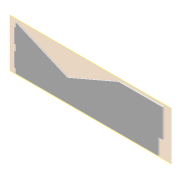
# Autodesk Inventor part: Frontal
Saved by Autodesk Inventor 2022 (Build 260153000, 153)
## iProperties
Created: 2022-06-06
Part Number: Frontal
Material: Generic
Document SubType Name: Modeling
Designer: ADMIN
Density: 1 g/cm^3
Appearance: Default
Author: ADMIN
Autodesk Inventor part; units mm, degrees
ref_plane "YZ Plane" through (0, 0, 0) normal (1, 0, 0) x (0, 1, 0)
ref_plane "XZ Plane" through (0, 0, 0) normal (0, 1, 0) x (-1, 0, 0)
ref_plane "XY Plane" through (0, 0, 0) normal (0, 0, 1) x (1, 0, 0)
ref_plane "Work Plane1" through (-2241.136, -81.6179, 0) normal (0, 0, 1) x (1, 0, 0)
sketch "Sketch1" plane through (-2241.136, -81.6179, 0) normal (0, 0, 1) x (1, 0, 0)
  line L0 (2006.136, 61.2134) -> (2006.136, 6.6179) projected
  line L1 (2006.136, 6.6179) -> (2476.136, 6.6179) projected
  line L2 (2476.136, 6.6179) -> (2476.136, 61.2134) projected
  line L3 (2476.136, 61.2134) -> (2491.136, 61.2134) projected
  line L4 (2491.136, 61.2134) -> (2491.136, 156.6179) projected
  line L5 (2491.136, 156.6179) -> (2341.136, 156.6179) projected
  line L6 (2341.136, 156.6179) -> (2166.136, 81.6179) projected
  line L7 (2166.136, 81.6179) -> (1991.136, 156.6179) projected
  line L8 (1991.136, 156.6179) -> (1991.136, 61.2134) projected
  line L9 (1991.136, 61.2134) -> (2006.136, 61.2134) projected
  line L10 (1991.136, 91.6179) -> (1991.136, 141.6179) projected
  line L11 (1991.136, 141.6179) -> (1986.136, 141.6179) projected
  line L12 (1986.136, 91.6179) -> (1986.136, 141.6179) projected
  line L13 (1991.136, 91.6179) -> (1986.136, 91.6179) projected
  line L14 (1991.136, 21.6179) -> (1991.136, 71.6179) projected
  line L15 (1991.136, 71.6179) -> (1986.136, 71.6179) projected
  line L16 (1986.136, 21.6179) -> (1986.136, 71.6179) projected
  line L17 (1991.136, 21.6179) -> (1986.136, 21.6179) projected
  line L18 (1986.136, 91.6179) -> (1991.136, 91.6179)
  line L19 (1991.136, 91.6179) -> (1991.136, 71.6179)
  line L20 (1991.136, 71.6179) -> (1986.136, 71.6179)
  line L21 (1986.136, 71.6179) -> (1986.136, 91.6179)
  line L22 (1991.136, 156.6179) -> (1986.136, 156.6179)
  line L23 (1986.136, 156.6179) -> (1986.136, 141.6179)
  line L24 (1986.136, 141.6179) -> (1991.136, 141.6179)
  line L25 (1991.136, 141.6179) -> (1991.136, 156.6179)
  line L26 (1986.136, 21.6179) -> (1991.136, 21.6179)
  line L27 (1991.136, 21.6179) -> (1991.136, 6.6179)
  line L28 (1991.136, 6.6179) -> (1986.136, 6.6179)
  line L29 (1986.136, 6.6179) -> (1986.136, 21.6179)
  line L30 (2006.136, 6.6179) -> (1991.136, 6.6179)
  line L31 (1991.136, 6.6179) -> (1991.136, 61.2134)
  line L32 (1991.136, 61.2134) -> (2006.136, 61.2134)
  line L33 (2006.136, 61.2134) -> (2006.136, 6.6179)
  line L34 (2496.136, 91.6179) -> (2496.136, 141.6179) projected
  line L35 (2496.136, 141.6179) -> (2491.136, 141.6179) projected
  line L36 (2491.136, 91.6179) -> (2491.136, 141.6179) projected
  line L37 (2496.136, 91.6179) -> (2491.136, 91.6179) projected
  line L38 (2496.136, 21.6179) -> (2496.136, 71.6179) projected
  line L39 (2496.136, 71.6179) -> (2491.136, 71.6179) projected
  line L40 (2491.136, 21.6179) -> (2491.136, 71.6179) projected
  line L41 (2496.136, 21.6179) -> (2491.136, 21.6179) projected
  line L42 (2491.136, 6.6179) -> (2476.136, 6.6179)
  line L43 (2476.136, 6.6179) -> (2476.136, 61.2134)
  line L44 (2476.136, 61.2134) -> (2491.136, 61.2134)
  line L45 (2491.136, 61.2134) -> (2491.136, 6.6179)
  point P0 (2241.136, 81.6179)
  point P1 (1991.136, 6.6179)
  point P2 (820.3787, 21.6179)
  point P3 (1320.3787, 21.6179)
  point P4 (820.3787, 20.4045)
  point P5 (1905.7573, 6.6179)
  point P6 (1305.3787, -34.1911)
  point P7 (820.3787, 21.6179)
  point P8 (2476.136, 6.6179)
  constraints: 40 end point, 10 parallel, 5 horizontal, 5 perpendicular, 1 point on line
extrude "Extrusion1" add sketch "Sketch1" along normal blind 5 contours L9 L8 L7 L6 L5 L4 L3 L2 L1 L0 | L0 L30 L27 L14 L9 | L14 L17 L16 L15 L8 | L2 L3 L40 L45 L42 | L13 L12 L11 L8 | L4 L39 L38 L41 L40 | L4 L35 L34 L37
sketch "Sketch2" plane through (-2241.136, -81.6179, 5) normal (0, 0, 1) x (1, 0, 0)
  line L0 (1991.136, 6.6179) -> (2491.136, 6.6179) projected
  line L1 (2491.136, 6.6179) -> (2491.136, 21.6179) projected
  line L2 (2491.136, 21.6179) -> (2496.136, 21.6179) projected
  line L3 (2496.136, 21.6179) -> (2496.136, 71.6179) projected
  line L4 (2496.136, 71.6179) -> (2491.136, 71.6179) projected
  line L5 (2491.136, 71.6179) -> (2491.136, 91.6179) projected
  line L6 (2491.136, 91.6179) -> (2496.136, 91.6179) projected
  line L7 (2496.136, 91.6179) -> (2496.136, 141.6179) projected
  line L8 (2496.136, 141.6179) -> (2491.136, 141.6179) projected
  line L9 (2491.136, 141.6179) -> (2491.136, 156.6179) projected
  line L10 (2491.136, 156.6179) -> (2341.136, 156.6179) projected
  line L11 (2341.136, 156.6179) -> (2166.136, 81.6179) projected
  line L12 (2166.136, 81.6179) -> (1991.136, 156.6179) projected
  line L13 (1991.136, 156.6179) -> (1991.136, 141.6179) projected
  line L14 (1991.136, 141.6179) -> (1986.136, 141.6179) projected
  line L15 (1986.136, 141.6179) -> (1986.136, 91.6179) projected
  line L16 (1986.136, 91.6179) -> (1991.136, 91.6179) projected
  line L17 (1991.136, 91.6179) -> (1991.136, 71.6179) projected
  line L18 (1991.136, 71.6179) -> (1986.136, 71.6179) projected
  line L19 (1986.136, 71.6179) -> (1986.136, 21.6179) projected
  line L20 (1986.136, 21.6179) -> (1991.136, 21.6179) projected
  line L21 (1991.136, 21.6179) -> (1991.136, 6.6179) projected
  line L22 (2371.136, 156.6179) -> (2401.136, 156.6179)
  line L23 (2401.136, 156.6179) -> (2401.136, 151.6179)
  line L24 (2401.136, 151.6179) -> (2371.136, 151.6179)
  line L25 (2371.136, 151.6179) -> (2371.136, 156.6179)
  line L26 (2431.136, 156.6179) -> (2461.136, 156.6179)
  line L27 (2461.136, 156.6179) -> (2461.136, 151.6179)
  line L28 (2461.136, 151.6179) -> (2431.136, 151.6179)
  line L29 (2431.136, 151.6179) -> (2431.136, 156.6179)
  line L30 (2166.136, 81.6179) -> (1991.136, 156.6179) projected
  line L31 (2037.4557, 136.7666) -> (2035.4861, 132.1708)
  line L32 (2035.4861, 132.1708) -> (2063.0604, 120.3533)
  line L33 (2063.0604, 120.3533) -> (2065.03, 124.949)
  line L34 (2092.6044, 113.1314) -> (2090.6348, 108.5357)
  line L35 (2090.6348, 108.5357) -> (2118.2091, 96.7181)
  line L36 (2118.2091, 96.7181) -> (2120.1787, 101.3138)
  line L37 (2166.136, 81.6179) -> (2166.136, 154.1179)
  line L38 (2294.8163, 136.7666) -> (2296.7859, 132.1708)
  line L39 (2296.7859, 132.1708) -> (2269.2115, 120.3533)
  line L40 (2269.2115, 120.3533) -> (2267.2419, 124.949)
  line L41 (2239.6676, 113.1314) -> (2241.6372, 108.5357)
  line L42 (2241.6372, 108.5357) -> (2214.0628, 96.7181)
  line L43 (2214.0628, 96.7181) -> (2212.0932, 101.3138)
  point P0 (2241.136, 81.6179)
  point P1 (2294.8163, 136.7666)
  point P2 (2267.2419, 124.949)
  point P3 (2239.6676, 113.1314)
  point P4 (2092.6044, 113.1314)
  point P5 (2037.4557, 136.7666)
  dimension "d2" = 30
  dimension "d3" = 5
  dimension "d4" = 30
  dimension "d5" = 5
  dimension "d6" = 30
  dimension "d7" = 30
  dimension "d10" = 30
  dimension "d11" = 5
  dimension "d12" = 30
  dimension "d13" = 5
  dimension "d14" = 30
  dimension "d15" = 50
  constraints: 42 end point, 8 perpendicular, 8 symmetric about line, 6 point on line, 4 parallel, 2 horizontal, 1 vertical
  measures "d2" distance of L23.end L24.end
  measures "d3" distance of L22.end L23.end
  measures "d4" distance of L27.end L28.end
  measures "d5" distance of L26.end L27.end
  measures "d6" distance from line of L29 L22.end
  measures "d7" distance between parallel lines of L9 L27
  measures "d10" distance of L31.end L32.end
  measures "d11" distance of L34.start L34.end
  measures "d12" distance of L34.end L35.end
  measures "d13" distance between parallel lines of L30 L32
  measures "d14" distance between parallel lines of L34 L33
  measures "d15" distance from line of L11.end L36
extrude "Extrusion2" cut sketch "Sketch2" against normal blind 5 contours L12 L33 L32 L31 | L27 L28 L29 L10 | L12 L36 L35 L34 | L23 L24 L25 L10 | L11 L41 L42 L43 | L38 L39 L40 L11
sketch "Sketch3" plane through (-2241.136, -81.6179, 5) normal (0, 0, 1) x (1, 0, 0)
  point P0 (2241.136, 81.6179)
sketch "Sketch4" plane through (-2241.136, -81.6179, 5) normal (0, 0, 1) x (1, 0, 0)
  line L0 (2371.136, 91.6179) -> (2401.136, 91.6179)
  line L1 (2401.136, 91.6179) -> (2401.136, 86.6179)
  line L2 (2401.136, 86.6179) -> (2371.136, 86.6179)
  line L3 (2371.136, 86.6179) -> (2371.136, 91.6179)
  line L4 (2214.0628, 96.7181) -> (2212.0932, 101.3138) projected
  line L5 (2212.0932, 101.3138) -> (2166.136, 81.6179) projected
  line L6 (2166.136, 81.6179) -> (2120.1787, 101.3138) projected
  line L7 (2120.1787, 101.3138) -> (2118.2091, 96.7181) projected
  line L8 (2118.2091, 96.7181) -> (2090.6348, 108.5357) projected
  line L9 (2090.6348, 108.5357) -> (2092.6044, 113.1314) projected
  line L10 (2092.6044, 113.1314) -> (2065.03, 124.949) projected
  line L11 (2065.03, 124.949) -> (2063.0604, 120.3533) projected
  line L12 (2063.0604, 120.3533) -> (2035.4861, 132.1708) projected
  line L13 (2035.4861, 132.1708) -> (2037.4557, 136.7666) projected
  line L14 (2037.4557, 136.7666) -> (1991.136, 156.6179) projected
  line L15 (1991.136, 156.6179) -> (1991.136, 141.6179) projected
  line L16 (1991.136, 141.6179) -> (1986.136, 141.6179) projected
  line L17 (1986.136, 141.6179) -> (1986.136, 91.6179) projected
  line L18 (1986.136, 91.6179) -> (1991.136, 91.6179) projected
  line L19 (1991.136, 91.6179) -> (1991.136, 71.6179) projected
  line L20 (1991.136, 71.6179) -> (1986.136, 71.6179) projected
  line L21 (1986.136, 71.6179) -> (1986.136, 21.6179) projected
  line L22 (1986.136, 21.6179) -> (1991.136, 21.6179) projected
  line L23 (1991.136, 21.6179) -> (1991.136, 6.6179) projected
  line L24 (1991.136, 6.6179) -> (2491.136, 6.6179) projected
  line L25 (2491.136, 6.6179) -> (2491.136, 21.6179) projected
  line L26 (2491.136, 21.6179) -> (2496.136, 21.6179) projected
  line L27 (2496.136, 21.6179) -> (2496.136, 71.6179) projected
  line L28 (2496.136, 71.6179) -> (2491.136, 71.6179) projected
  line L29 (2491.136, 71.6179) -> (2491.136, 91.6179) projected
  line L30 (2491.136, 91.6179) -> (2496.136, 91.6179) projected
  line L31 (2496.136, 91.6179) -> (2496.136, 141.6179) projected
  line L32 (2496.136, 141.6179) -> (2491.136, 141.6179) projected
  line L33 (2491.136, 141.6179) -> (2491.136, 156.6179) projected
  line L34 (2491.136, 156.6179) -> (2461.136, 156.6179) projected
  line L35 (2461.136, 156.6179) -> (2461.136, 151.6179) projected
  line L36 (2461.136, 151.6179) -> (2431.136, 151.6179) projected
  line L37 (2431.136, 151.6179) -> (2431.136, 156.6179) projected
  line L38 (2431.136, 156.6179) -> (2401.136, 156.6179) projected
  line L39 (2401.136, 156.6179) -> (2401.136, 151.6179) projected
  line L40 (2401.136, 151.6179) -> (2371.136, 151.6179) projected
  line L41 (2371.136, 151.6179) -> (2371.136, 156.6179) projected
  line L42 (2371.136, 156.6179) -> (2341.136, 156.6179) projected
  line L43 (2341.136, 156.6179) -> (2294.8163, 136.7666) projected
  line L44 (2294.8163, 136.7666) -> (2296.7859, 132.1708) projected
  line L45 (2296.7859, 132.1708) -> (2269.2115, 120.3533) projected
  line L46 (2269.2115, 120.3533) -> (2267.2419, 124.949) projected
  line L47 (2267.2419, 124.949) -> (2239.6676, 113.1314) projected
  line L48 (2239.6676, 113.1314) -> (2241.6372, 108.5357) projected
  line L49 (2241.6372, 108.5357) -> (2214.0628, 96.7181) projected
  line L50 (2431.136, 91.6179) -> (2461.136, 91.6179)
  line L51 (2461.136, 91.6179) -> (2461.136, 86.6179)
  line L52 (2461.136, 86.6179) -> (2431.136, 86.6179)
  line L53 (2431.136, 86.6179) -> (2431.136, 91.6179)
  point P0 (2241.136, 81.6179)
  dimension "d16" = 30
  dimension "d17" = 5
  dimension "d18" = 80
  dimension "d19" = 30
  dimension "d20" = 5
  dimension "d21" = 30
  dimension "d22" = 30
  constraints: 16 end point, 4 parallel, 2 horizontal, 2 perpendicular
  measures "d16" distance of L1.end L2.end
  measures "d17" distance of L0.end L1.end
  measures "d18" distance between parallel lines of L24 L2
  measures "d19" distance of L51.end L52.end
  measures "d20" distance of L50.end L51.end
  measures "d21" distance of L0.end L50.start
  measures "d22" distance between parallel lines of L29 L51
extrude "Extrusion3" cut sketch "Sketch4" against normal blind 5 contours L0 L1 L2 L3 | L50 L51 L52 L53
body "Solid1"
